Autodesk Inventor part; units mm, degrees
(part 2 of 4)
  spline S23 degree 5 poles (-0.775, -5.2999) (-0.7753, -5.3017) (-0.7759, -5.3054) (-0.7769, -5.3109) (-0.7785, -5.3181) (-0.7807, -5.3272) (-0.7831, -5.3361) (-0.7857, -5.3451) (-0.7884, -5.354) (-0.7911, -5.363) (-0.7939, -5.3719) (-0.7968, -5.3808) (-0.7998, -5.3897) (-0.8029, -5.3986) (-0.8061, -5.4075) (-0.8093, -5.4163) (-0.8127, -5.4252) (-0.8162, -5.434) (-0.8197, -5.4428) (-0.8232, -5.4516) (-0.8269, -5.4604) (-0.8306, -5.4691) (-0.8343, -5.4779) (-0.8382, -5.4866) (-0.8421, -5.4954) (-0.846, -5.5041) (-0.8501, -5.5128) (-0.8541, -5.5215) (-0.8583, -5.5302) (-0.8625, -5.5388) (-0.8667, -5.5475) (-0.8711, -5.5561) (-0.8754, -5.5648) (-0.8798, -5.5734) (-0.8843, -5.582) (-0.8888, -5.5906) (-0.8934, -5.5992) (-0.898, -5.6078) (-0.9027, -5.6163) (-0.9075, -5.6249) (-0.9122, -5.6334) (-0.9171, -5.6419) (-0.9219, -5.6504) (-0.9269, -5.6589) (-0.9318, -5.6674) (-0.9369, -5.6759) (-0.9419, -5.6844) (-0.947, -5.6928) (-0.9522, -5.7013) (-0.9574, -5.7097) (-0.9627, -5.7181) (-0.968, -5.7265) (-0.9733, -5.7349) (-0.9787, -5.7433) (-0.9841, -5.7517) (-0.9896, -5.7601) (-0.9951, -5.7684) (-1.0007, -5.7767) (-1.0063, -5.7851) (-1.0119, -5.7934) (-1.0176, -5.8017) (-1.0233, -5.81) (-1.0291, -5.8183) (-1.0349, -5.8265) (-1.0408, -5.8348) (-1.0467, -5.843) (-1.0526, -5.8512) (-1.0586, -5.8595) (-1.067, -5.8709) (-1.0743, -5.8808) (-1.0804, -5.8889) (-1.0853, -5.8954) (-1.0891, -5.9003) knots 0 0 0 0 0 0 0.014286 0.028571 0.042857 0.057143 0.071429 0.085714 0.1 0.114286 0.128571 0.142857 0.157143 0.171429 0.185714 0.2 0.214286 0.228571 0.242857 0.257143 0.271429 0.285714 0.3 0.314286 0.328571 0.342857 0.357143 0.371429 0.385714 0.4 0.414286 0.428571 0.442857 0.457143 0.471429 0.485714 0.5 0.514286 0.528571 0.542857 0.557143 0.571429 0.585714 0.6 0.614286 0.628571 0.642857 0.657143 0.671429 0.685714 0.7 0.714286 0.728571 0.742857 0.757143 0.771429 0.785714 0.8 0.814286 0.828571 0.842857 0.857143 0.871429 0.885714 0.9 0.914286 0.928571 0.942857 0.957143 1 1 1 1 1 1
  line L23 (-0.7648, -5.2336) -> (-0.775, -5.2999)
  arc A24 (-0.7648, -5.2336) -> (-0.4836, -5.267) centre (0, 0) ccw
  line L24 (-0.4836, -5.267) -> (-0.4892, -5.3339)
  spline S24 degree 5 poles (-0.4892, -5.3339) (-0.4894, -5.3357) (-0.4896, -5.3394) (-0.4899, -5.345) (-0.4901, -5.3524) (-0.4901, -5.3617) (-0.4898, -5.371) (-0.4894, -5.3803) (-0.4889, -5.3896) (-0.4883, -5.399) (-0.4877, -5.4083) (-0.487, -5.4177) (-0.4862, -5.427) (-0.4852, -5.4364) (-0.4842, -5.4457) (-0.4831, -5.4551) (-0.4819, -5.4645) (-0.4806, -5.4739) (-0.4793, -5.4833) (-0.4779, -5.4926) (-0.4764, -5.502) (-0.4749, -5.5114) (-0.4733, -5.5208) (-0.4716, -5.5302) (-0.4698, -5.5396) (-0.468, -5.549) (-0.4662, -5.5584) (-0.4642, -5.5678) (-0.4622, -5.5772) (-0.4602, -5.5867) (-0.4581, -5.5961) (-0.4559, -5.6055) (-0.4537, -5.6149) (-0.4514, -5.6243) (-0.4491, -5.6337) (-0.4467, -5.6432) (-0.4443, -5.6526) (-0.4418, -5.662) (-0.4392, -5.6714) (-0.4366, -5.6808) (-0.434, -5.6903) (-0.4313, -5.6997) (-0.4286, -5.7091) (-0.4258, -5.7185) (-0.4229, -5.7279) (-0.42, -5.7374) (-0.4171, -5.7468) (-0.4141, -5.7562) (-0.4111, -5.7656) (-0.408, -5.775) (-0.4048, -5.7845) (-0.4017, -5.7939) (-0.3984, -5.8033) (-0.3952, -5.8127) (-0.3918, -5.8221) (-0.3885, -5.8315) (-0.3851, -5.8409) (-0.3816, -5.8503) (-0.3781, -5.8598) (-0.3746, -5.8692) (-0.371, -5.8786) (-0.3674, -5.888) (-0.3637, -5.8974) (-0.36, -5.9068) (-0.3563, -5.9161) (-0.3525, -5.9255) (-0.3486, -5.9349) (-0.3447, -5.9443) (-0.3392, -5.9575) (-0.3345, -5.9687) (-0.3304, -5.9781) (-0.3272, -5.9856) (-0.3247, -5.9912) knots 0 0 0 0 0 0 0.014286 0.028571 0.042857 0.057143 0.071429 0.085714 0.1 0.114286 0.128571 0.142857 0.157143 0.171429 0.185714 0.2 0.214286 0.228571 0.242857 0.257143 0.271429 0.285714 0.3 0.314286 0.328571 0.342857 0.357143 0.371429 0.385714 0.4 0.414286 0.428571 0.442857 0.457143 0.471429 0.485714 0.5 0.514286 0.528571 0.542857 0.557143 0.571429 0.585714 0.6 0.614286 0.628571 0.642857 0.657143 0.671429 0.685714 0.7 0.714286 0.728571 0.742857 0.757143 0.771429 0.785714 0.8 0.814286 0.828571 0.842857 0.857143 0.871429 0.885714 0.9 0.914286 0.928571 0.942857 0.957143 1 1 1 1 1 1
  arc A25 (-0.3247, -5.9912) -> (-0.103, -5.9991) centre (0, 0) ccw
  spline S25 degree 5 poles (0.1079, -5.3552) (0.1079, -5.357) (0.1079, -5.3607) (0.1078, -5.3663) (0.1075, -5.3737) (0.1068, -5.383) (0.1059, -5.3922) (0.1048, -5.4015) (0.1036, -5.4108) (0.1024, -5.42) (0.1011, -5.4293) (0.0997, -5.4386) (0.0982, -5.4479) (0.0966, -5.4571) (0.095, -5.4664) (0.0932, -5.4757) (0.0913, -5.4849) (0.0894, -5.4942) (0.0874, -5.5035) (0.0853, -5.5127) (0.0831, -5.522) (0.0809, -5.5312) (0.0787, -5.5405) (0.0763, -5.5498) (0.0739, -5.559) (0.0714, -5.5683) (0.0689, -5.5775) (0.0663, -5.5868) (0.0636, -5.596) (0.0609, -5.6052) (0.0582, -5.6145) (0.0553, -5.6237) (0.0525, -5.633) (0.0495, -5.6422) (0.0465, -5.6514) (0.0435, -5.6606) (0.0404, -5.6699) (0.0372, -5.6791) (0.034, -5.6883) (0.0307, -5.6975) (0.0274, -5.7067) (0.0241, -5.7159) (0.0207, -5.7251) (0.0172, -5.7343) (0.0137, -5.7435) (0.0101, -5.7527) (0.0065, -5.7619) (0.0029, -5.7711) (-0.0008, -5.7803) (-0.0046, -5.7894) (-0.0084, -5.7986) (-0.0122, -5.8078) (-0.0161, -5.8169) (-0.02, -5.8261) (-0.024, -5.8352) (-0.028, -5.8444) (-0.0321, -5.8535) (-0.0362, -5.8627) (-0.0404, -5.8718) (-0.0446, -5.8809) (-0.0488, -5.8901) (-0.0531, -5.8992) (-0.0574, -5.9083) (-0.0618, -5.9174) (-0.0662, -5.9265) (-0.0707, -5.9356) (-0.0752, -5.9447) (-0.0797, -5.9538) (-0.0861, -5.9665) (-0.0917, -5.9774) (-0.0964, -5.9864) (-0.1002, -5.9937) (-0.103, -5.9991) knots 0 0 0 0 0 0 0.014286 0.028571 0.042857 0.057143 0.071429 0.085714 0.1 0.114286 0.128571 0.142857 0.157143 0.171429 0.185714 0.2 0.214286 0.228571 0.242857 0.257143 0.271429 0.285714 0.3 0.314286 0.328571 0.342857 0.357143 0.371429 0.385714 0.4 0.414286 0.428571 0.442857 0.457143 0.471429 0.485714 0.5 0.514286 0.528571 0.542857 0.557143 0.571429 0.585714 0.6 0.614286 0.628571 0.642857 0.657143 0.671429 0.685714 0.7 0.714286 0.728571 0.742857 0.757143 0.771429 0.785714 0.8 0.814286 0.828571 0.842857 0.857143 0.871429 0.885714 0.9 0.914286 0.928571 0.942857 0.957143 1 1 1 1 1 1
  line L25 (0.107, -5.2881) -> (0.1079, -5.3552)
  arc A26 (0.107, -5.2881) -> (0.39, -5.2748) centre (0, 0) ccw
  line L26 (0.39, -5.2748) -> (0.3954, -5.3416)
  spline S26 degree 5 poles (0.3954, -5.3416) (0.3955, -5.3435) (0.3959, -5.3472) (0.3965, -5.3527) (0.3975, -5.3601) (0.3991, -5.3692) (0.4009, -5.3784) (0.4029, -5.3875) (0.4049, -5.3966) (0.407, -5.4057) (0.4092, -5.4148) (0.4114, -5.4239) (0.4137, -5.433) (0.4162, -5.4421) (0.4187, -5.4512) (0.4214, -5.4602) (0.4241, -5.4693) (0.4269, -5.4783) (0.4298, -5.4874) (0.4327, -5.4964) (0.4357, -5.5054) (0.4388, -5.5144) (0.4419, -5.5234) (0.4451, -5.5324) (0.4484, -5.5414) (0.4517, -5.5504) (0.4551, -5.5593) (0.4585, -5.5683) (0.4621, -5.5773) (0.4656, -5.5862) (0.4693, -5.5951) (0.4729, -5.6041) (0.4767, -5.613) (0.4805, -5.6219) (0.4843, -5.6308) (0.4882, -5.6397) (0.4922, -5.6486) (0.4962, -5.6575) (0.5002, -5.6664) (0.5044, -5.6752) (0.5085, -5.6841) (0.5127, -5.6929) (0.517, -5.7018) (0.5213, -5.7106) (0.5256, -5.7194) (0.53, -5.7282) (0.5345, -5.7371) (0.539, -5.7459) (0.5435, -5.7546) (0.5481, -5.7634) (0.5528, -5.7722) (0.5575, -5.781) (0.5622, -5.7897) (0.567, -5.7985) (0.5718, -5.8072) (0.5766, -5.8159) (0.5816, -5.8247) (0.5865, -5.8334) (0.5915, -5.8421) (0.5965, -5.8508) (0.6016, -5.8594) (0.6067, -5.8681) (0.6119, -5.8768) (0.6171, -5.8854) (0.6224, -5.8941) (0.6277, -5.9027) (0.633, -5.9114) (0.6384, -5.92) (0.646, -5.932) (0.6525, -5.9424) (0.658, -5.9509) (0.6625, -5.9578) (0.6659, -5.9629) knots 0 0 0 0 0 0 0.014286 0.028571 0.042857 0.057143 0.071429 0.085714 0.1 0.114286 0.128571 0.142857 0.157143 0.171429 0.185714 0.2 0.214286 0.228571 0.242857 0.257143 0.271429 0.285714 0.3 0.314286 0.328571 0.342857 0.357143 0.371429 0.385714 0.4 0.414286 0.428571 0.442857 0.457143 0.471429 0.485714 0.5 0.514286 0.528571 0.542857 0.557143 0.571429 0.585714 0.6 0.614286 0.628571 0.642857 0.657143 0.671429 0.685714 0.7 0.714286 0.728571 0.742857 0.757143 0.771429 0.785714 0.8 0.814286 0.828571 0.842857 0.857143 0.871429 0.885714 0.9 0.914286 0.928571 0.942857 0.957143 1 1 1 1 1 1
  arc A27 (0.6659, -5.9629) -> (0.8858, -5.9343) centre (0, 0) ccw
  spline S27 degree 5 poles (0.9879, -5.2644) (0.9882, -5.2662) (0.9888, -5.2699) (0.9896, -5.2754) (0.9905, -5.2828) (0.9913, -5.292) (0.9919, -5.3013) (0.9924, -5.3106) (0.9928, -5.3199) (0.9931, -5.3293) (0.9933, -5.3386) (0.9935, -5.348) (0.9936, -5.3574) (0.9935, -5.3668) (0.9934, -5.3762) (0.9932, -5.3857) (0.9929, -5.3951) (0.9925, -5.4046) (0.992, -5.414) (0.9915, -5.4235) (0.9909, -5.433) (0.9902, -5.4425) (0.9895, -5.452) (0.9887, -5.4615) (0.9879, -5.471) (0.987, -5.4806) (0.986, -5.4901) (0.985, -5.4997) (0.9839, -5.5092) (0.9827, -5.5188) (0.9815, -5.5283) (0.9802, -5.5379) (0.9789, -5.5475) (0.9775, -5.5571) (0.9761, -5.5667) (0.9746, -5.5763) (0.973, -5.5859) (0.9715, -5.5955) (0.9698, -5.6051) (0.9681, -5.6147) (0.9664, -5.6244) (0.9646, -5.634) (0.9627, -5.6436) (0.9608, -5.6533) (0.9589, -5.6629) (0.9569, -5.6726) (0.9548, -5.6822) (0.9527, -5.6919) (0.9506, -5.7016) (0.9484, -5.7112) (0.9462, -5.7209) (0.9439, -5.7306) (0.9416, -5.7402) (0.9392, -5.7499) (0.9368, -5.7596) (0.9343, -5.7693) (0.9318, -5.779) (0.9293, -5.7887) (0.9267, -5.7984) (0.924, -5.8081) (0.9213, -5.8178) (0.9186, -5.8275) (0.9158, -5.8372) (0.913, -5.8469) (0.9102, -5.8566) (0.9073, -5.8663) (0.9043, -5.876) (0.9013, -5.8857) (0.8971, -5.8993) (0.8934, -5.9109) (0.8903, -5.9207) (0.8877, -5.9284) (0.8858, -5.9343) knots 0 0 0 0 0 0 0.014286 0.028571 0.042857 0.057143 0.071429 0.085714 0.1 0.114286 0.128571 0.142857 0.157143 0.171429 0.185714 0.2 0.214286 0.228571 0.242857 0.257143 0.271429 0.285714 0.3 0.314286 0.328571 0.342857 0.357143 0.371429 0.385714 0.4 0.414286 0.428571 0.442857 0.457143 0.471429 0.485714 0.5 0.514286 0.528571 0.542857 0.557143 0.571429 0.585714 0.6 0.614286 0.628571 0.642857 0.657143 0.671429 0.685714 0.7 0.714286 0.728571 0.742857 0.757143 0.771429 0.785714 0.8 0.814286 0.828571 0.842857 0.857143 0.871429 0.885714 0.9 0.914286 0.928571 0.942857 0.957143 1 1 1 1 1 1
  line L27 (0.976, -5.1984) -> (0.9879, -5.2644)
  arc A28 (0.976, -5.1984) -> (1.2528, -5.1387) centre (0, 0) ccw
  line L28 (1.2528, -5.1387) -> (1.2692, -5.2037)
  spline S28 degree 5 poles (1.2692, -5.2037) (1.2697, -5.2055) (1.2706, -5.2091) (1.2721, -5.2145) (1.2744, -5.2216) (1.2774, -5.2303) (1.2807, -5.239) (1.2841, -5.2477) (1.2876, -5.2563) (1.2912, -5.265) (1.2948, -5.2736) (1.2985, -5.2822) (1.3023, -5.2908) (1.3062, -5.2994) (1.3102, -5.3079) (1.3143, -5.3164) (1.3185, -5.3249) (1.3228, -5.3333) (1.3271, -5.3418) (1.3315, -5.3502) (1.3359, -5.3586) (1.3404, -5.367) (1.345, -5.3753) (1.3496, -5.3837) (1.3543, -5.392) (1.3591, -5.4003) (1.3639, -5.4086) (1.3688, -5.4169) (1.3737, -5.4251) (1.3787, -5.4334) (1.3838, -5.4416) (1.3889, -5.4498) (1.394, -5.458) (1.3993, -5.4662) (1.4045, -5.4743) (1.4098, -5.4824) (1.4152, -5.4906) (1.4206, -5.4987) (1.4261, -5.5067) (1.4316, -5.5148) (1.4371, -5.5229) (1.4428, -5.5309) (1.4484, -5.5389) (1.4541, -5.5469) (1.4599, -5.5549) (1.4657, -5.5629) (1.4715, -5.5708) (1.4774, -5.5788) (1.4833, -5.5867) (1.4893, -5.5946) (1.4953, -5.6025) (1.5014, -5.6104) (1.5075, -5.6182) (1.5136, -5.6261) (1.5198, -5.6339) (1.5261, -5.6417) (1.5323, -5.6495) (1.5387, -5.6573) (1.545, -5.665) (1.5514, -5.6728) (1.5579, -5.6805) (1.5643, -5.6882) (1.5709, -5.6959) (1.5774, -5.7036) (1.584, -5.7113) (1.5907, -5.7189) (1.5973, -5.7266) (1.6041, -5.7342) (1.6135, -5.7448) (1.6217, -5.7539) (1.6286, -5.7615) (1.6341, -5.7675) (1.6382, -5.772) knots 0 0 0 0 0 0 0.014286 0.028571 0.042857 0.057143 0.071429 0.085714 0.1 0.114286 0.128571 0.142857 0.157143 0.171429 0.185714 0.2 0.214286 0.228571 0.242857 0.257143 0.271429 0.285714 0.3 0.314286 0.328571 0.342857 0.357143 0.371429 0.385714 0.4 0.414286 0.428571 0.442857 0.457143 0.471429 0.485714 0.5 0.514286 0.528571 0.542857 0.557143 0.571429 0.585714 0.6 0.614286 0.628571 0.642857 0.657143 0.671429 0.685714 0.7 0.714286 0.728571 0.742857 0.757143 0.771429 0.785714 0.8 0.814286 0.828571 0.842857 0.857143 0.871429 0.885714 0.9 0.914286 0.928571 0.942857 0.957143 1 1 1 1 1 1
  arc A29 (1.6382, -5.772) -> (1.8505, -5.7075) centre (0, 0) ccw
  spline S29 degree 5 poles (1.8409, -5.03) (1.8415, -5.0317) (1.8427, -5.0352) (1.8444, -5.0405) (1.8465, -5.0477) (1.8489, -5.0567) (1.851, -5.0657) (1.853, -5.0748) (1.8549, -5.084) (1.8567, -5.0931) (1.8585, -5.1023) (1.8602, -5.1115) (1.8618, -5.1208) (1.8633, -5.1301) (1.8648, -5.1394) (1.8661, -5.1487) (1.8673, -5.1581) (1.8685, -5.1675) (1.8696, -5.1769) (1.8706, -5.1863) (1.8716, -5.1958) (1.8725, -5.2053) (1.8734, -5.2148) (1.8742, -5.2243) (1.8749, -5.2338) (1.8756, -5.2434) (1.8762, -5.2529) (1.8767, -5.2625) (1.8772, -5.2721) (1.8777, -5.2818) (1.878, -5.2914) (1.8784, -5.301) (1.8786, -5.3107) (1.8788, -5.3204) (1.879, -5.3301) (1.8791, -5.3398) (1.8792, -5.3495) (1.8792, -5.3593) (1.8791, -5.3691) (1.8791, -5.3788) (1.8789, -5.3886) (1.8787, -5.3984) (1.8785, -5.4082) (1.8782, -5.418) (1.8779, -5.4279) (1.8775, -5.4377) (1.8771, -5.4476) (1.8766, -5.4575) (1.8761, -5.4673) (1.8755, -5.4772) (1.8749, -5.4871) (1.8742, -5.497) (1.8735, -5.507) (1.8728, -5.5169) (1.872, -5.5269) (1.8712, -5.5368) (1.8703, -5.5468) (1.8694, -5.5568) (1.8684, -5.5668) (1.8674, -5.5768) (1.8663, -5.5868) (1.8652, -5.5968) (1.8641, -5.6068) (1.8629, -5.6168) (1.8617, -5.6269) (1.8605, -5.6369) (1.8591, -5.647) (1.8578, -5.6571) (1.8559, -5.6712) (1.8541, -5.6833) (1.8526, -5.6934) (1.8514, -5.7015) (1.8505, -5.7075) knots 0 0 0 0 0 0 0.014286 0.028571 0.042857 0.057143 0.071429 0.085714 0.1 0.114286 0.128571 0.142857 0.157143 0.171429 0.185714 0.2 0.214286 0.228571 0.242857 0.257143 0.271429 0.285714 0.3 0.314286 0.328571 0.342857 0.357143 0.371429 0.385714 0.4 0.414286 0.428571 0.442857 0.457143 0.471429 0.485714 0.5 0.514286 0.528571 0.542857 0.557143 0.571429 0.585714 0.6 0.614286 0.628571 0.642857 0.657143 0.671429 0.685714 0.7 0.714286 0.728571 0.742857 0.757143 0.771429 0.785714 0.8 0.814286 0.828571 0.842857 0.857143 0.871429 0.885714 0.9 0.914286 0.928571 0.942857 0.957143 1 1 1 1 1 1
  line L29 (1.8183, -4.9668) -> (1.8409, -5.03)
  arc A30 (1.8183, -4.9668) -> (2.0816, -4.8624) centre (0, 0) ccw
  line L30 (2.0816, -4.8624) -> (2.1084, -4.9238)
  spline S30 degree 5 poles (2.1084, -4.9238) (2.1091, -4.9255) (2.1107, -4.9289) (2.113, -4.934) (2.1164, -4.9406) (2.1209, -4.9487) (2.1255, -4.9568) (2.1303, -4.9648) (2.1352, -4.9727) (2.1402, -4.9807) (2.1452, -4.9886) (2.1503, -4.9965) (2.1554, -5.0043) (2.1607, -5.0121) (2.166, -5.0199) (2.1715, -5.0276) (2.177, -5.0352) (2.1826, -5.0429) (2.1882, -5.0505) (2.1939, -5.0581) (2.1997, -5.0656) (2.2055, -5.0732) (2.2114, -5.0807) (2.2174, -5.0881) (2.2234, -5.0956) (2.2294, -5.103) (2.2356, -5.1104) (2.2417, -5.1177) (2.248, -5.125) (2.2542, -5.1323) (2.2606, -5.1396) (2.267, -5.1469) (2.2734, -5.1541) (2.2799, -5.1613) (2.2864, -5.1685) (2.293, -5.1756) (2.2996, -5.1827) (2.3063, -5.1898) (2.313, -5.1969) (2.3198, -5.204) (2.3266, -5.211) (2.3334, -5.218) (2.3403, -5.225) (2.3473, -5.2319) (2.3543, -5.2389) (2.3613, -5.2458) (2.3684, -5.2527) (2.3755, -5.2595) (2.3826, -5.2664) (2.3898, -5.2732) (2.3971, -5.28) (2.4043, -5.2867) (2.4116, -5.2935) (2.419, -5.3002) (2.4264, -5.3069) (2.4338, -5.3136) (2.4413, -5.3202) (2.4488, -5.3269) (2.4564, -5.3335) (2.464, -5.3401) (2.4716, -5.3466) (2.4792, -5.3532) (2.4869, -5.3597) (2.4947, -5.3662) (2.5025, -5.3727) (2.5103, -5.3791) (2.5181, -5.3855) (2.526, -5.3919) (2.5371, -5.4009) (2.5466, -5.4085) (2.5547, -5.4148) (2.5611, -5.4199) (2.5659, -5.4236) knots 0 0 0 0 0 0 0.014286 0.028571 0.042857 0.057143 0.071429 0.085714 0.1 0.114286 0.128571 0.142857 0.157143 0.171429 0.185714 0.2 0.214286 0.228571 0.242857 0.257143 0.271429 0.285714 0.3 0.314286 0.328571 0.342857 0.357143 0.371429 0.385714 0.4 0.414286 0.428571 0.442857 0.457143 0.471429 0.485714 0.5 0.514286 0.528571 0.542857 0.557143 0.571429 0.585714 0.6 0.614286 0.628571 0.642857 0.657143 0.671429 0.685714 0.7 0.714286 0.728571 0.742857 0.757143 0.771429 0.785714 0.8 0.814286 0.828571 0.842857 0.857143 0.871429 0.885714 0.9 0.914286 0.928571 0.942857 0.957143 1 1 1 1 1 1
  arc A31 (2.5659, -5.4236) -> (2.7646, -5.3251) centre (0, 0) ccw
  spline S31 degree 5 poles (2.6437, -4.6584) (2.6446, -4.66) (2.6464, -4.6633) (2.6489, -4.6682) (2.6522, -4.6749) (2.6559, -4.6834) (2.6595, -4.692) (2.663, -4.7006) (2.6664, -4.7093) (2.6697, -4.7181) (2.6729, -4.7268) (2.6762, -4.7356) (2.6793, -4.7445) (2.6823, -4.7534) (2.6852, -4.7624) (2.6881, -4.7714) (2.6909, -4.7804) (2.6936, -4.7895) (2.6962, -4.7986) (2.6988, -4.8077) (2.7013, -4.8169) (2.7038, -4.8261) (2.7062, -4.8353) (2.7085, -4.8445) (2.7108, -4.8538) (2.713, -4.8631) (2.7152, -4.8725) (2.7173, -4.8819) (2.7194, -4.8912) (2.7214, -4.9007) (2.7234, -4.9101) (2.7253, -4.9196) (2.7271, -4.9291) (2.7289, -4.9386) (2.7307, -4.9481) (2.7324, -4.9577) (2.7341, -4.9673) (2.7357, -4.9769) (2.7372, -4.9865) (2.7388, -4.9962) (2.7402, -5.0059) (2.7417, -5.0155) (2.743, -5.0253) (2.7444, -5.035) (2.7457, -5.0448) (2.7469, -5.0545) (2.7481, -5.0643) (2.7493, -5.0741) (2.7504, -5.084) (2.7514, -5.0938) (2.7525, -5.1037) (2.7535, -5.1136) (2.7544, -5.1235) (2.7553, -5.1334) (2.7562, -5.1434) (2.757, -5.1533) (2.7577, -5.1633) (2.7585, -5.1733) (2.7592, -5.1833) (2.7598, -5.1933) (2.7604, -5.2034) (2.761, -5.2134) (2.7615, -5.2235) (2.762, -5.2336) (2.7625, -5.2437) (2.7629, -5.2538) (2.7633, -5.264) (2.7636, -5.2741) (2.764, -5.2884) (2.7643, -5.3006) (2.7645, -5.3108) (2.7646, -5.319) (2.7646, -5.3251) knots 0 0 0 0 0 0 0.014286 0.028571 0.042857 0.057143 0.071429 0.085714 0.1 0.114286 0.128571 0.142857 0.157143 0.171429 0.185714 0.2 0.214286 0.228571 0.242857 0.257143 0.271429 0.285714 0.3 0.314286 0.328571 0.342857 0.357143 0.371429 0.385714 0.4 0.414286 0.428571 0.442857 0.457143 0.471429 0.485714 0.5 0.514286 0.528571 0.542857 0.557143 0.571429 0.585714 0.6 0.614286 0.628571 0.642857 0.657143 0.671429 0.685714 0.7 0.714286 0.728571 0.742857 0.757143 0.771429 0.785714 0.8 0.814286 0.828571 0.842857 0.857143 0.871429 0.885714 0.9 0.914286 0.928571 0.942857 0.957143 1 1 1 1 1 1
  line L31 (2.611, -4.5998) -> (2.6437, -4.6584)
  arc A32 (2.611, -4.5998) -> (2.8535, -4.4534) centre (0, 0) ccw
  line L32 (2.8535, -4.4534) -> (2.8901, -4.5096)
  spline S32 degree 5 poles (2.8901, -4.5096) (2.8911, -4.5112) (2.8932, -4.5143) (2.8963, -4.5189) (2.9007, -4.5249) (2.9065, -4.5322) (2.9124, -4.5393) (2.9185, -4.5464) (2.9246, -4.5534) (2.9308, -4.5605) (2.937, -4.5674) (2.9433, -4.5744) (2.9497, -4.5813) (2.9562, -4.5881) (2.9627, -4.5949) (2.9694, -4.6016) (2.9761, -4.6082) (2.9828, -4.6149) (2.9897, -4.6214) (2.9965, -4.628) (3.0035, -4.6345) (3.0105, -4.6409) (3.0175, -4.6474) (3.0246, -4.6538) (3.0317, -4.6601) (3.0389, -4.6664) (3.0462, -4.6727) (3.0535, -4.6789) (3.0609, -4.6851) (3.0683, -4.6913) (3.0757, -4.6974) (3.0832, -4.7035) (3.0907, -4.7096) (3.0983, -4.7156) (3.1059, -4.7216) (3.1136, -4.7276) (3.1213, -4.7336) (3.129, -4.7395) (3.1368, -4.7453) (3.1447, -4.7512) (3.1525, -4.757) (3.1605, -4.7628) (3.1684, -4.7685) (3.1764, -4.7742) (3.1844, -4.7799) (3.1925, -4.7856) (3.2006, -4.7912) (3.2088, -4.7968) (3.2169, -4.8024) (3.2252, -4.8079) (3.2334, -4.8134) (3.2417, -4.8189) (3.25, -4.8243) (3.2584, -4.8298) (3.2668, -4.8351) (3.2752, -4.8405) (3.2837, -4.8458) (3.2922, -4.8511) (3.3007, -4.8564) (3.3093, -4.8617) (3.3179, -4.8669) (3.3265, -4.8721) (3.3352, -4.8772) (3.3439, -4.8824) (3.3526, -4.8875) (3.3614, -4.8926) (3.3702, -4.8976) (3.379, -4.9026) (3.3914, -4.9096) (3.4021, -4.9156) (3.4111, -4.9205) (3.4183, -4.9244) (3.4237, -4.9273) knots 0 0 0 0 0 0 0.014286 0.028571 0.042857 0.057143 0.071429 0.085714 0.1 0.114286 0.128571 0.142857 0.157143 0.171429 0.185714 0.2 0.214286 0.228571 0.242857 0.257143 0.271429 0.285714 0.3 0.314286 0.328571 0.342857 0.357143 0.371429 0.385714 0.4 0.414286 0.428571 0.442857 0.457143 0.471429 0.485714 0.5 0.514286 0.528571 0.542857 0.557143 0.571429 0.585714 0.6 0.614286 0.628571 0.642857 0.657143 0.671429 0.685714 0.7 0.714286 0.728571 0.742857 0.757143 0.771429 0.785714 0.8 0.814286 0.828571 0.842857 0.857143 0.871429 0.885714 0.9 0.914286 0.928571 0.942857 0.957143 1 1 1 1 1 1
  arc A33 (3.4237, -4.9273) -> (3.6034, -4.7974) centre (0, 0) ccw
  spline S33 degree 5 poles (3.3744, -4.1597) (3.3755, -4.1612) (3.3778, -4.1641) (3.3812, -4.1685) (3.3855, -4.1746) (3.3906, -4.1824) (3.3955, -4.1902) (3.4004, -4.1982) (3.4051, -4.2062) (3.4098, -4.2143) (3.4145, -4.2224) (3.4191, -4.2306) (3.4237, -4.2388) (3.4281, -4.2471) (3.4325, -4.2554) (3.4368, -4.2638) (3.441, -4.2723) (3.4451, -4.2808) (3.4492, -4.2894) (3.4533, -4.2979) (3.4573, -4.3066) (3.4612, -4.3152) (3.4651, -4.3239) (3.469, -4.3327) (3.4727, -4.3414) (3.4765, -4.3503) (3.4802, -4.3591) (3.4838, -4.368) (3.4874, -4.3769) (3.4909, -4.3859) (3.4944, -4.3949) (3.4978, -4.4039) (3.5012, -4.413) (3.5046, -4.4221) (3.5079, -4.4312) (3.5111, -4.4403) (3.5144, -4.4495) (3.5175, -4.4587) (3.5207, -4.468) (3.5237, -4.4773) (3.5268, -4.4866) (3.5298, -4.4959) (3.5328, -4.5052) (3.5357, -4.5146) (3.5386, -4.524) (3.5414, -4.5335) (3.5442, -4.5429) (3.5469, -4.5524) (3.5497, -4.5619) (3.5523, -4.5715) (3.555, -4.581) (3.5576, -4.5906) (3.5601, -4.6003) (3.5627, -4.6099) (3.5651, -4.6196) (3.5676, -4.6293) (3.57, -4.639) (3.5724, -4.6487) (3.5747, -4.6585) (3.577, -4.6682) (3.5792, -4.6781) (3.5815, -4.6879) (3.5836, -4.6977) (3.5858, -4.7076) (3.5879, -4.7175) (3.59, -4.7274) (3.592, -4.7374) (3.594, -4.7473) (3.5967, -4.7613) (3.599, -4.7733) (3.6009, -4.7833) (3.6023, -4.7914) (3.6034, -4.7974) knots 0 0 0 0 0 0 0.014286 0.028571 0.042857 0.057143 0.071429 0.085714 0.1 0.114286 0.128571 0.142857 0.157143 0.171429 0.185714 0.2 0.214286 0.228571 0.242857 0.257143 0.271429 0.285714 0.3 0.314286 0.328571 0.342857 0.357143 0.371429 0.385714 0.4 0.414286 0.428571 0.442857 0.457143 0.471429 0.485714 0.5 0.514286 0.528571 0.542857 0.557143 0.571429 0.585714 0.6 0.614286 0.628571 0.642857 0.657143 0.671429 0.685714 0.7 0.714286 0.728571 0.742857 0.757143 0.771429 0.785714 0.8 0.814286 0.828571 0.842857 0.857143 0.871429 0.885714 0.9 0.914286 0.928571 0.942857 0.957143 1 1 1 1 1 1
  line L33 (3.3325, -4.1073) -> (3.3744, -4.1597)
  arc A34 (3.3325, -4.1073) -> (3.5476, -3.923) centre (0, 0) ccw
  line L34 (3.5476, -3.923) -> (3.5929, -3.9724)
  spline S34 degree 5 poles (3.5929, -3.9724) (3.5942, -3.9738) (3.5967, -3.9765) (3.6006, -3.9805) (3.6059, -3.9857) (3.6128, -3.9919) (3.6198, -3.998) (3.627, -4.004) (3.6342, -4.01) (3.6414, -4.0159) (3.6487, -4.0217) (3.6561, -4.0275) (3.6635, -4.0333) (3.671, -4.039) (3.6786, -4.0446) (3.6863, -4.0501) (3.694, -4.0556) (3.7017, -4.061) (3.7095, -4.0663) (3.7174, -4.0716) (3.7253, -4.0769) (3.7333, -4.0821) (3.7413, -4.0873) (3.7493, -4.0925) (3.7574, -4.0976) (3.7656, -4.1026) (3.7738, -4.1076) (3.782, -4.1125) (3.7903, -4.1174) (3.7986, -4.1223) (3.8069, -4.1271) (3.8153, -4.1319) (3.8237, -4.1367) (3.8322, -4.1414) (3.8407, -4.146) (3.8493, -4.1507) (3.8578, -4.1552) (3.8665, -4.1598) (3.8751, -4.1643) (3.8838, -4.1688) (3.8925, -4.1732) (3.9013, -4.1776) (3.9101, -4.182) (3.9189, -4.1863) (3.9278, -4.1906) (3.9366, -4.1948) (3.9456, -4.199) (3.9545, -4.2032) (3.9635, -4.2074) (3.9725, -4.2115) (3.9816, -4.2156) (3.9907, -4.2196) (3.9998, -4.2236) (4.0089, -4.2276) (4.0181, -4.2315) (4.0273, -4.2354) (4.0365, -4.2393) (4.0458, -4.2431) (4.0551, -4.2469) (4.0644, -4.2507) (4.0737, -4.2544) (4.0831, -4.2581) (4.0925, -4.2618) (4.1019, -4.2654) (4.1114, -4.269) (4.1208, -4.2726) (4.1304, -4.2761) (4.1399, -4.2796) (4.1533, -4.2845) (4.1648, -4.2886) (4.1744, -4.2919) (4.1822, -4.2946) (4.188, -4.2966) knots 0 0 0 0 0 0 0.014286 0.028571 0.042857 0.057143 0.071429 0.085714 0.1 0.114286 0.128571 0.142857 0.157143 0.171429 0.185714 0.2 0.214286 0.228571 0.242857 0.257143 0.271429 0.285714 0.3 0.314286 0.328571 0.342857 0.357143 0.371429 0.385714 0.4 0.414286 0.428571 0.442857 0.457143 0.471429 0.485714 0.5 0.514286 0.528571 0.542857 0.557143 0.571429 0.585714 0.6 0.614286 0.628571 0.642857 0.657143 0.671429 0.685714 0.7 0.714286 0.728571 0.742857 0.757143 0.771429 0.785714 0.8 0.814286 0.828571 0.842857 0.857143 0.871429 0.885714 0.9 0.914286 0.928571 0.942857 0.957143 1 1 1 1 1 1
  arc A35 (4.188, -4.2966) -> (4.3439, -4.1389) centre (0, 0) ccw
  spline S35 degree 5 poles (4.013, -3.5476) (4.0144, -3.5488) (4.0171, -3.5513) (4.0212, -3.5552) (4.0264, -3.5604) (4.0327, -3.5672) (4.0389, -3.5742) (4.045, -3.5813) (4.051, -3.5884) (4.057, -3.5956) (4.0629, -3.6028) (4.0688, -3.6101) (4.0746, -3.6175) (4.0804, -3.6249) (4.0861, -3.6324) (4.0917, -3.64) (4.0972, -3.6477) (4.1027, -3.6554) (4.1082, -3.6631) (4.1136, -3.6709) (4.119, -3.6788) (4.1243, -3.6867) (4.1296, -3.6946) (4.1348, -3.7026) (4.14, -3.7106) (4.1451, -3.7187) (4.1502, -3.7269) (4.1552, -3.735) (4.1602, -3.7432) (4.1652, -3.7515) (4.1701, -3.7598) (4.175, -3.7681) (4.1798, -3.7765) (4.1846, -3.7849) (4.1894, -3.7934) (4.1941, -3.8019) (4.1988, -3.8104) (4.2034, -3.819) (4.208, -3.8276) (4.2126, -3.8362) (4.2172, -3.8449) (4.2216, -3.8536) (4.2261, -3.8623) (4.2305, -3.8711) (4.2349, -3.8799) (4.2393, -3.8887) (4.2436, -3.8976) (4.2479, -3.9065) (4.2521, -3.9155) (4.2563, -3.9244) (4.2605, -3.9334) (4.2646, -3.9425) (4.2688, -3.9515) (4.2728, -3.9606) (4.2769, -3.9698) (4.2809, -3.9789) (4.2848, -3.9881) (4.2888, -3.9973) (4.2927, -4.0066) (4.2966, -4.0158) (4.3004, -4.0251) (4.3042, -4.0345) (4.308, -4.0438) (4.3117, -4.0532) (4.3154, -4.0626) (4.3191, -4.0721) (4.3227, -4.0815) (4.3264, -4.091) (4.3314, -4.1043) (4.3356, -4.1158) (4.3391, -4.1254) (4.3418, -4.1331) (4.3439, -4.1389) knots 0 0 0 0 0 0 0.014286 0.028571 0.042857 0.057143 0.071429 0.085714 0.1 0.114286 0.128571 0.142857 0.157143 0.171429 0.185714 0.2 0.214286 0.228571 0.242857 0.257143 0.271429 0.285714 0.3 0.314286 0.328571 0.342857 0.357143 0.371429 0.385714 0.4 0.414286 0.428571 0.442857 0.457143 0.471429 0.485714 0.5 0.514286 0.528571 0.542857 0.557143 0.571429 0.585714 0.6 0.614286 0.628571 0.642857 0.657143 0.671429 0.685714 0.7 0.714286 0.728571 0.742857 0.757143 0.771429 0.785714 0.8 0.814286 0.828571 0.842857 0.857143 0.871429 0.885714 0.9 0.914286 0.928571 0.942857 0.957143 1 1 1 1 1 1
  line L35 (3.9631, -3.5028) -> (4.013, -3.5476)
  arc A36 (3.9631, -3.5028) -> (4.1449, -3.2856) centre (0, 0) ccw
  line L36 (4.1449, -3.2856) -> (4.1978, -3.3269)
  spline S36 degree 5 poles (4.1978, -3.3269) (4.1992, -3.328) (4.2022, -3.3303) (4.2067, -3.3336) (4.2128, -3.3378) (4.2206, -3.3429) (4.2285, -3.3477) (4.2365, -3.3524) (4.2446, -3.3571) (4.2528, -3.3617) (4.2609, -3.3663) (4.2691, -3.3708) (4.2774, -3.3753) (4.2858, -3.3797) (4.2941, -3.3839) (4.3026, -3.3881) (4.3111, -3.3922) (4.3197, -3.3963) (4.3283, -3.4003) (4.3369, -3.4042) (4.3455, -3.4081) (4.3543, -3.412) (4.363, -3.4158) (4.3718, -3.4195) (4.3806, -3.4232) (4.3895, -3.4268) (4.3984, -3.4304) (4.4073, -3.4339) (4.4163, -3.4374) (4.4253, -3.4409) (4.4343, -3.4442) (4.4434, -3.4476) (4.4525, -3.4509) (4.4616, -3.4541) (4.4707, -3.4573) (4.4799, -3.4605) (4.4892, -3.4636) (4.4984, -3.4667) (4.5077, -3.4697) (4.517, -3.4727) (4.5263, -3.4756) (4.5357, -3.4785) (4.5451, -3.4814) (4.5545, -3.4842) (4.5639, -3.4869) (4.5734, -3.4897) (4.5829, -3.4924) (4.5924, -3.495) (4.602, -3.4976) (4.6115, -3.5002) (4.6211, -3.5027) (4.6308, -3.5052) (4.6404, -3.5077) (4.6501, -3.5101) (4.6598, -3.5124) (4.6695, -3.5148) (4.6792, -3.5171) (4.689, -3.5193) (4.6988, -3.5215) (4.7086, -3.5237) (4.7184, -3.5259) (4.7283, -3.528) (4.7381, -3.53) (4.748, -3.5321) (4.7579, -3.5341) (4.7679, -3.536) (4.7778, -3.5379) (4.7878, -3.5398) (4.8018, -3.5424) (4.8139, -3.5446) (4.8239, -3.5463) (4.832, -3.5477) (4.8381, -3.5487) knots 0 0 0 0 0 0 0.014286 0.028571 0.042857 0.057143 0.071429 0.085714 0.1 0.114286 0.128571 0.142857 0.157143 0.171429 0.185714 0.2 0.214286 0.228571 0.242857 0.257143 0.271429 0.285714 0.3 0.314286 0.328571 0.342857 0.357143 0.371429 0.385714 0.4 0.414286 0.428571 0.442857 0.457143 0.471429 0.485714 0.5 0.514286 0.528571 0.542857 0.557143 0.571429 0.585714 0.6 0.614286 0.628571 0.642857 0.657143 0.671429 0.685714 0.7 0.714286 0.728571 0.742857 0.757143 0.771429 0.785714 0.8 0.814286 0.828571 0.842857 0.857143 0.871429 0.885714 0.9 0.914286 0.928571 0.942857 0.957143 1 1 1 1 1 1
  arc A37 (4.8381, -3.5487) -> (4.9659, -3.3675) centre (0, 0) ccw
  spline S37 degree 5 poles (4.5422, -2.8387) (4.5437, -2.8397) (4.5469, -2.8417) (4.5515, -2.8448) (4.5575, -2.8492) (4.5649, -2.8548) (4.5721, -2.8607) (4.5793, -2.8666) (4.5864, -2.8727) (4.5935, -2.8788) (4.6005, -2.8849) (4.6075, -2.8912) (4.6145, -2.8975) (4.6214, -2.9039) (4.6282, -2.9103) (4.635, -2.9169) (4.6418, -2.9235) (4.6484, -2.9302) (4.6551, -2.937) (4.6617, -2.9438) (4.6683, -2.9506) (4.6748, -2.9575) (4.6814, -2.9645) (4.6878, -2.9715) (4.6943, -2.9786) (4.7006, -2.9857) (4.707, -2.9929) (4.7133, -3.0002) (4.7196, -3.0074) (4.7259, -3.0148) (4.7321, -3.0221) (4.7383, -3.0296) (4.7444, -3.037) (4.7505, -3.0445) (4.7566, -3.0521) (4.7627, -3.0597) (4.7687, -3.0673) (4.7747, -3.075) (4.7807, -3.0827) (4.7866, -3.0905) (4.7925, -3.0983) (4.7984, -3.1062) (4.8042, -3.114) (4.81, -3.122) (4.8158, -3.1299) (4.8215, -3.1379) (4.8272, -3.146) (4.8329, -3.1541) (4.8386, -3.1622) (4.8442, -3.1703) (4.8498, -3.1785) (4.8554, -3.1868) (4.8609, -3.195) (4.8665, -3.2033) (4.8719, -3.2117) (4.8774, -3.22) (4.8828, -3.2284) (4.8882, -3.2369) (4.8936, -3.2454) (4.8989, -3.2539) (4.9043, -3.2624) (4.9096, -3.271) (4.9148, -3.2796) (4.92, -3.2882) (4.9253, -3.2969) (4.9304, -3.3056) (4.9356, -3.3144) (4.9407, -3.3231) (4.9478, -3.3355) (4.9539, -3.3461) (4.9589, -3.355) (4.9629, -3.3621) (4.9659, -3.3675) knots 0 0 0 0 0 0 0.014286 0.028571 0.042857 0.057143 0.071429 0.085714 0.1 0.114286 0.128571 0.142857 0.157143 0.171429 0.185714 0.2 0.214286 0.228571 0.242857 0.257143 0.271429 0.285714 0.3 0.314286 0.328571 0.342857 0.357143 0.371429 0.385714 0.4 0.414286 0.428571 0.442857 0.457143 0.471429 0.485714 0.5 0.514286 0.528571 0.542857 0.557143 0.571429 0.585714 0.6 0.614286 0.628571 0.642857 0.657143 0.671429 0.685714 0.7 0.714286 0.728571 0.742857 0.757143 0.771429 0.785714 0.8 0.814286 0.828571 0.842857 0.857143 0.871429 0.885714 0.9 0.914286 0.928571 0.942857 0.957143 1 1 1 1 1 1
  line L37 (4.4856, -2.8027) -> (4.5422, -2.8387)
  arc A38 (4.4856, -2.8027) -> (4.6292, -2.5586) centre (0, 0) ccw
  line L38 (4.6292, -2.5586) -> (4.6881, -2.5906)
  spline S38 degree 5 poles (4.6881, -2.5906) (4.6897, -2.5915) (4.693, -2.5932) (4.698, -2.5957) (4.7047, -2.5989) (4.7132, -2.6026) (4.7219, -2.6061) (4.7306, -2.6094) (4.7393, -2.6127) (4.7481, -2.6159) (4.7569, -2.6191) (4.7657, -2.6222) (4.7746, -2.6252) (4.7836, -2.6281) (4.7926, -2.631) (4.8016, -2.6337) (4.8107, -2.6364) (4.8198, -2.639) (4.8289, -2.6415) (4.8381, -2.644) (4.8472, -2.6464) (4.8565, -2.6488) (4.8657, -2.6511) (4.875, -2.6533) (4.8843, -2.6555) (4.8936, -2.6576) (4.903, -2.6597) (4.9124, -2.6617) (4.9218, -2.6636) (4.9313, -2.6656) (4.9407, -2.6674) (4.9502, -2.6692) (4.9597, -2.671) (4.9693, -2.6727) (4.9788, -2.6743) (4.9884, -2.6759) (4.998, -2.6775) (5.0076, -2.679) (5.0173, -2.6804) (5.027, -2.6818) (5.0367, -2.6832) (5.0464, -2.6845) (5.0561, -2.6858) (5.0658, -2.687) (5.0756, -2.6882) (5.0854, -2.6893) (5.0952, -2.6904) (5.105, -2.6915) (5.1149, -2.6925) (5.1248, -2.6934) (5.1346, -2.6943) (5.1445, -2.6952) (5.1544, -2.696) (5.1644, -2.6968) (5.1743, -2.6976) (5.1843, -2.6983) (5.1943, -2.6989) (5.2043, -2.6995) (5.2143, -2.7001) (5.2243, -2.7007) (5.2344, -2.7012) (5.2445, -2.7016) (5.2545, -2.702) (5.2646, -2.7024) (5.2747, -2.7027) (5.2849, -2.703) (5.295, -2.7033) (5.3052, -2.7035) (5.3194, -2.7037) (5.3316, -2.7039) (5.3418, -2.704) (5.35, -2.704) (5.3562, -2.704) knots 0 0 0 0 0 0 0.014286 0.028571 0.042857 0.057143 0.071429 0.085714 0.1 0.114286 0.128571 0.142857 0.157143 0.171429 0.185714 0.2 0.214286 0.228571 0.242857 0.257143 0.271429 0.285714 0.3 0.314286 0.328571 0.342857 0.357143 0.371429 0.385714 0.4 0.414286 0.428571 0.442857 0.457143 0.471429 0.485714 0.5 0.514286 0.528571 0.542857 0.557143 0.571429 0.585714 0.6 0.614286 0.628571 0.642857 0.657143 0.671429 0.685714 0.7 0.714286 0.728571 0.742857 0.757143 0.771429 0.785714 0.8 0.814286 0.828571 0.842857 0.857143 0.871429 0.885714 0.9 0.914286 0.928571 0.942857 0.957143 1 1 1 1 1 1
  arc A39 (5.3562, -2.704) -> (5.4524, -2.5042) centre (0, 0) ccw
  spline S39 degree 5 poles (4.9475, -2.0523) (4.9492, -2.0531) (4.9526, -2.0545) (4.9576, -2.0569) (4.9643, -2.0602) (4.9725, -2.0645) (4.9806, -2.0691) (4.9886, -2.0738) (4.9966, -2.0786) (5.0046, -2.0835) (5.0126, -2.0884) (5.0206, -2.0934) (5.0285, -2.0984) (5.0363, -2.1036) (5.0441, -2.1089) (5.0519, -2.1142) (5.0596, -2.1196) (5.0673, -2.1252) (5.075, -2.1307) (5.0827, -2.1363) (5.0903, -2.142) (5.0979, -2.1478) (5.1054, -2.1536) (5.113, -2.1594) (5.1205, -2.1653) (5.128, -2.1713) (5.1354, -2.1774) (5.1428, -2.1835) (5.1502, -2.1896) (5.1576, -2.1958) (5.165, -2.2021) (5.1723, -2.2083) (5.1796, -2.2147) (5.1869, -2.2211) (5.1941, -2.2275) (5.2013, -2.234) (5.2085, -2.2406) (5.2157, -2.2472) (5.2229, -2.2538) (5.23, -2.2605) (5.2371, -2.2672) (5.2442, -2.274) (5.2512, -2.2808) (5.2583, -2.2877) (5.2653, -2.2946) (5.2723, -2.3016) (5.2792, -2.3085) (5.2862, -2.3156) (5.2931, -2.3227) (5.3, -2.3298) (5.3068, -2.3369) (5.3137, -2.3441) (5.3205, -2.3514) (5.3273, -2.3586) (5.3341, -2.366) (5.3409, -2.3733) (5.3476, -2.3807) (5.3543, -2.3882) (5.361, -2.3956) (5.3677, -2.4031) (5.3743, -2.4107) (5.381, -2.4183) (5.3876, -2.4259) (5.3942, -2.4336) (5.4007, -2.4413) (5.4073, -2.449) (5.4138, -2.4568) (5.4203, -2.4646) (5.4294, -2.4756) (5.4371, -2.4851) (5.4435, -2.493) (5.4486, -2.4994) (5.4524, -2.5042) knots 0 0 0 0 0 0 0.014286 0.028571 0.042857 0.057143 0.071429 0.085714 0.1 0.114286 0.128571 0.142857 0.157143 0.171429 0.185714 0.2 0.214286 0.228571 0.242857 0.257143 0.271429 0.285714 0.3 0.314286 0.328571 0.342857 0.357143 0.371429 0.385714 0.4 0.414286 0.428571 0.442857 0.457143 0.471429 0.485714 0.5 0.514286 0.528571 0.542857 0.557143 0.571429 0.585714 0.6 0.614286 0.628571 0.642857 0.657143 0.671429 0.685714 0.7 0.714286 0.728571 0.742857 0.757143 0.771429 0.785714 0.8 0.814286 0.828571 0.842857 0.857143 0.871429 0.885714 0.9 0.914286 0.928571 0.942857 0.957143 1 1 1 1 1 1
  line L39 (4.8857, -2.0262) -> (4.9475, -2.0523)
  arc A40 (4.8857, -2.0262) -> (4.9872, -1.7617) centre (0, 0) ccw
  line L40 (4.9872, -1.7617) -> (5.0506, -1.7836)
  spline S40 degree 5 poles (5.0506, -1.7836) (5.0523, -1.7842) (5.0558, -1.7854) (5.0612, -1.7871) (5.0683, -1.7891) (5.0773, -1.7913) (5.0864, -1.7933) (5.0955, -1.7952) (5.1047, -1.797) (5.1139, -1.7987) (5.1231, -1.8004) (5.1323, -1.802) (5.1416, -1.8035) (5.1509, -1.805) (5.1602, -1.8063) (5.1696, -1.8075) (5.179, -1.8086) (5.1884, -1.8097) (5.1978, -1.8107) (5.2073, -1.8116) (5.2167, -1.8125) (5.2262, -1.8133) (5.2357, -1.814) (5.2452, -1.8147) (5.2548, -1.8154) (5.2643, -1.8159) (5.2739, -1.8164) (5.2835, -1.8168) (5.2931, -1.8172) (5.3027, -1.8175) (5.3124, -1.8178) (5.322, -1.818) (5.3317, -1.8182) (5.3414, -1.8183) (5.3511, -1.8183) (5.3608, -1.8183) (5.3705, -1.8183) (5.3803, -1.8182) (5.39, -1.818) (5.3998, -1.8178) (5.4096, -1.8176) (5.4194, -1.8173) (5.4292, -1.8169) (5.439, -1.8165) (5.4489, -1.8161) (5.4587, -1.8156) (5.4685, -1.8151) (5.4784, -1.8145) (5.4883, -1.8138) (5.4982, -1.8132) (5.5081, -1.8124) (5.518, -1.8117) (5.5279, -1.8109) (5.5378, -1.81) (5.5478, -1.8091) (5.5577, -1.8082) (5.5677, -1.8072) (5.5776, -1.8061) (5.5876, -1.805) (5.5976, -1.8039) (5.6076, -1.8028) (5.6176, -1.8016) (5.6276, -1.8003) (5.6376, -1.799) (5.6477, -1.7977) (5.6577, -1.7963) (5.6677, -1.7949) (5.6778, -1.7934) (5.6919, -1.7913) (5.704, -1.7895) (5.714, -1.7878) (5.7221, -1.7865) (5.7282, -1.7855) knots 0 0 0 0 0 0 0.014286 0.028571 0.042857 0.057143 0.071429 0.085714 0.1 0.114286 0.128571 0.142857 0.157143 0.171429 0.185714 0.2 0.214286 0.228571 0.242857 0.257143 0.271429 0.285714 0.3 0.314286 0.328571 0.342857 0.357143 0.371429 0.385714 0.4 0.414286 0.428571 0.442857 0.457143 0.471429 0.485714 0.5 0.514286 0.528571 0.542857 0.557143 0.571429 0.585714 0.6 0.614286 0.628571 0.642857 0.657143 0.671429 0.685714 0.7 0.714286 0.728571 0.742857 0.757143 0.771429 0.785714 0.8 0.814286 0.828571 0.842857 0.857143 0.871429 0.885714 0.9 0.914286 0.928571 0.942857 0.957143 1 1 1 1 1 1
  arc A41 (5.7282, -1.7855) -> (5.7902, -1.5726) centre (0, 0) ccw
  spline S41 degree 5 poles (5.2178, -1.21) (5.2196, -1.2105) (5.2232, -1.2114) (5.2286, -1.2128) (5.2357, -1.215) (5.2445, -1.2179) (5.2532, -1.2211) (5.2619, -1.2244) (5.2706, -1.2278) (5.2793, -1.2313) (5.288, -1.2348) (5.2966, -1.2385) (5.3053, -1.2422) (5.3139, -1.246) (5.3225, -1.2499) (5.331, -1.2539) (5.3395, -1.2579) (5.348, -1.2621) (5.3565, -1.2663) (5.365, -1.2706) (5.3734, -1.275) (5.3819, -1.2794) (5.3903, -1.2839) (5.3987, -1.2884) (5.4071, -1.293) (5.4154, -1.2977) (5.4238, -1.3024) (5.4321, -1.3072) (5.4404, -1.312) (5.4487, -1.3169) (5.457, -1.3219) (5.4652, -1.3269) (5.4735, -1.332) (5.4817, -1.3371) (5.4899, -1.3422) (5.4981, -1.3475) (5.5063, -1.3527) (5.5144, -1.3581) (5.5226, -1.3634) (5.5307, -1.3689) (5.5388, -1.3743) (5.5469, -1.3798) (5.555, -1.3854) (5.5631, -1.391) (5.5711, -1.3967) (5.5792, -1.4024) (5.5872, -1.4081) (5.5952, -1.4139) (5.6032, -1.4198) (5.6112, -1.4256) (5.6191, -1.4316) (5.6271, -1.4376) (5.635, -1.4436) (5.6429, -1.4496) (5.6508, -1.4557) (5.6587, -1.4619) (5.6665, -1.4681) (5.6744, -1.4743) (5.6822, -1.4806) (5.69, -1.4869) (5.6978, -1.4932) (5.7056, -1.4996) (5.7134, -1.5061) (5.7212, -1.5125) (5.7289, -1.519) (5.7366, -1.5256) (5.7443, -1.5322) (5.752, -1.5388) (5.7628, -1.5482) (5.772, -1.5562) (5.7796, -1.563) (5.7857, -1.5685) (5.7902, -1.5726) knots 0 0 0 0 0 0 0.014286 0.028571 0.042857 0.057143 0.071429 0.085714 0.1 0.114286 0.128571 0.142857 0.157143 0.171429 0.185714 0.2 0.214286 0.228571 0.242857 0.257143 0.271429 0.285714 0.3 0.314286 0.328571 0.342857 0.357143 0.371429 0.385714 0.4 0.414286 0.428571 0.442857 0.457143 0.471429 0.485714 0.5 0.514286 0.528571 0.542857 0.557143 0.571429 0.585714 0.6 0.614286 0.628571 0.642857 0.657143 0.671429 0.685714 0.7 0.714286 0.728571 0.742857 0.757143 0.771429 0.785714 0.8 0.814286 0.828571 0.842857 0.857143 0.871429 0.885714 0.9 0.914286 0.928571 0.942857 0.957143 1 1 1 1 1 1
  line L41 (5.1526, -1.1944) -> (5.2178, -1.21)
  arc A42 (5.1526, -1.1944) -> (5.2091, -0.9169) centre (0, 0) ccw
  line L42 (5.2091, -0.9169) -> (5.2752, -0.928)
  spline S42 degree 5 poles (5.2752, -0.928) (5.2771, -0.9283) (5.2808, -0.9289) (5.2863, -0.9296) (5.2937, -0.9305) (5.3029, -0.9312) (5.3122, -0.9317) (5.3215, -0.932) (5.3308, -0.9323) (5.3402, -0.9325) (5.3496, -0.9326) (5.3589, -0.9327) (5.3683, -0.9327) (5.3777, -0.9325) (5.3872, -0.9323) (5.3966, -0.9319) (5.406, -0.9315) (5.4155, -0.931) (5.4249, -0.9304) (5.4344, -0.9298) (5.4439, -0.9291) (5.4534, -0.9284) (5.4629, -0.9275) (5.4724, -0.9266) (5.4819, -0.9257) (5.4914, -0.9247) (5.501, -0.9236) (5.5105, -0.9224) (5.52, -0.9212) (5.5296, -0.9199) (5.5391, -0.9186) (5.5487, -0.9173) (5.5583, -0.9158) (5.5678, -0.9143) (5.5774, -0.9128) (5.587, -0.9112) (5.5966, -0.9095) (5.6062, -0.9078) (5.6158, -0.9061) (5.6254, -0.9043) (5.635, -0.9024) (5.6446, -0.9005) (5.6542, -0.8985) (5.6638, -0.8965) (5.6735, -0.8945) (5.6831, -0.8924) (5.6927, -0.8902) (5.7023, -0.888) (5.712, -0.8858) (5.7216, -0.8835) (5.7313, -0.8811) (5.7409, -0.8787) (5.7506, -0.8763) (5.7602, -0.8738) (5.7699, -0.8713) (5.7795, -0.8687) (5.7892, -0.8661) (5.7988, -0.8634) (5.8085, -0.8607) (5.8182, -0.858) (5.8278, -0.8552) (5.8375, -0.8524) (5.8472, -0.8495) (5.8568, -0.8466) (5.8665, -0.8436) (5.8762, -0.8406) (5.8859, -0.8375) (5.8955, -0.8344) (5.9091, -0.83) (5.9207, -0.8262) (5.9304, -0.823) (5.9381, -0.8203) (5.9439, -0.8183) knots 0 0 0 0 0 0 0.014286 0.028571 0.042857 0.057143 0.071429 0.085714 0.1 0.114286 0.128571 0.142857 0.157143 0.171429 0.185714 0.2 0.214286 0.228571 0.242857 0.257143 0.271429 0.285714 0.3 0.314286 0.328571 0.342857 0.357143 0.371429 0.385714 0.4 0.414286 0.428571 0.442857 0.457143 0.471429 0.485714 0.5 0.514286 0.528571 0.542857 0.557143 0.571429 0.585714 0.6 0.614286 0.628571 0.642857 0.657143 0.671429 0.685714 0.7 0.714286 0.728571 0.742857 0.757143 0.771429 0.785714 0.8 0.814286 0.828571 0.842857 0.857143 0.871429 0.885714 0.9 0.914286 0.928571 0.942857 0.957143 1 1 1 1 1 1
  arc A43 (5.9439, -0.8183) -> (5.9701, -0.5981) centre (0, 0) ccw
  spline S43 degree 5 poles (5.3458, -0.3347) (5.3476, -0.3348) (5.3513, -0.3351) (5.3569, -0.3357) (5.3643, -0.3366) (5.3734, -0.3381) (5.3826, -0.3398) (5.3917, -0.3416) (5.4008, -0.3436) (5.41, -0.3456) (5.4191, -0.3476) (5.4282, -0.3498) (5.4374, -0.352) (5.4465, -0.3543) (5.4556, -0.3568) (5.4647, -0.3593) (5.4737, -0.3619) (5.4828, -0.3646) (5.4919, -0.3674) (5.5009, -0.3702) (5.51, -0.3731) (5.519, -0.3761) (5.5281, -0.3791) (5.5371, -0.3822) (5.5461, -0.3854) (5.5551, -0.3886) (5.5642, -0.3919) (5.5732, -0.3953) (5.5822, -0.3987) (5.5911, -0.4022) (5.6001, -0.4057) (5.6091, -0.4093) (5.6181, -0.4129) (5.627, -0.4166) (5.636, -0.4203) (5.6449, -0.4241) (5.6538, -0.428) (5.6628, -0.4319) (5.6717, -0.4358) (5.6806, -0.4399) (5.6895, -0.4439) (5.6984, -0.448) (5.7073, -0.4522) (5.7162, -0.4564) (5.725, -0.4606) (5.7339, -0.4649) (5.7428, -0.4693) (5.7516, -0.4737) (5.7604, -0.4781) (5.7693, -0.4826) (5.7781, -0.4872) (5.7869, -0.4918) (5.7957, -0.4964) (5.8045, -0.5011) (5.8133, -0.5058) (5.8221, -0.5106) (5.8309, -0.5154) (5.8397, -0.5202) (5.8484, -0.5251) (5.8572, -0.53) (5.8659, -0.535) (5.8746, -0.5401) (5.8834, -0.5451) (5.8921, -0.5502) (5.9008, -0.5554) (5.9095, -0.5606) (5.9182, -0.5658) (5.9269, -0.5711) (5.939, -0.5785) (5.9494, -0.585) (5.958, -0.5904) (5.9649, -0.5948) (5.9701, -0.5981) knots 0 0 0 0 0 0 0.014286 0.028571 0.042857 0.057143 0.071429 0.085714 0.1 0.114286 0.128571 0.142857 0.157143 0.171429 0.185714 0.2 0.214286 0.228571 0.242857 0.257143 0.271429 0.285714 0.3 0.314286 0.328571 0.342857 0.357143 0.371429 0.385714 0.4 0.414286 0.428571 0.442857 0.457143 0.471429 0.485714 0.5 0.514286 0.528571 0.542857 0.557143 0.571429 0.585714 0.6 0.614286 0.628571 0.642857 0.657143 0.671429 0.685714 0.7 0.714286 0.728571 0.742857 0.757143 0.771429 0.785714 0.8 0.814286 0.828571 0.842857 0.857143 0.871429 0.885714 0.9 0.914286 0.928571 0.942857 0.957143 1 1 1 1 1 1
  line L43 (5.2789, -0.33) -> (5.3458, -0.3347)
  arc A44 (5.2789, -0.33) -> (5.289, -0.047) centre (0, 0) ccw
  line L44 (5.289, -0.047) -> (5.356, -0.0471)
  spline S44 degree 5 poles (5.356, -0.0471) (5.3579, -0.0471) (5.3616, -0.047) (5.3672, -0.0469) (5.3746, -0.0465) (5.3839, -0.0456) (5.3931, -0.0446) (5.4023, -0.0434) (5.4116, -0.0421) (5.4208, -0.0408) (5.4301, -0.0394) (5.4394, -0.0379) (5.4486, -0.0363) (5.4579, -0.0347) (5.4671, -0.0329) (5.4764, -0.031) (5.4856, -0.029) (5.4949, -0.027) (5.5041, -0.0248) (5.5133, -0.0227) (5.5226, -0.0204) (5.5318, -0.0181) (5.541, -0.0157) (5.5503, -0.0133) (5.5595, -0.0108) (5.5687, -0.0082) (5.5779, -0.0055) (5.5872, -0.0028) (5.5964, -0.0001) (5.6056, 0.0027) (5.6148, 0.0056) (5.624, 0.0085) (5.6332, 0.0115) (5.6424, 0.0146) (5.6516, 0.0177) (5.6608, 0.0208) (5.67, 0.024) (5.6791, 0.0273) (5.6883, 0.0306) (5.6975, 0.034) (5.7067, 0.0374) (5.7158, 0.0409) (5.725, 0.0444) (5.7342, 0.0479) (5.7433, 0.0515) (5.7525, 0.0552) (5.7616, 0.0589) (5.7707, 0.0627) (5.7799, 0.0665) (5.789, 0.0703) (5.7981, 0.0742) (5.8073, 0.0782) (5.8164, 0.0822) (5.8255, 0.0862) (5.8346, 0.0903) (5.8437, 0.0944) (5.8528, 0.0986) (5.8619, 0.1028) (5.871, 0.1071) (5.88, 0.1114) (5.8891, 0.1157) (5.8982, 0.1201) (5.9073, 0.1245) (5.9163, 0.129) (5.9254, 0.1335) (5.9344, 0.1381) (5.9434, 0.1427) (5.9525, 0.1473) (5.9651, 0.1539) (5.9759, 0.1596) (5.985, 0.1644) (5.9922, 0.1683) (5.9976, 0.1712) knots 0 0 0 0 0 0 0.014286 0.028571 0.042857 0.057143 0.071429 0.085714 0.1 0.114286 0.128571 0.142857 0.157143 0.171429 0.185714 0.2 0.214286 0.228571 0.242857 0.257143 0.271429 0.285714 0.3 0.314286 0.328571 0.342857 0.357143 0.371429 0.385714 0.4 0.414286 0.428571 0.442857 0.457143 0.471429 0.485714 0.5 0.514286 0.528571 0.542857 0.557143 0.571429 0.585714 0.6 0.614286 0.628571 0.642857 0.657143 0.671429 0.685714 0.7 0.714286 0.728571 0.742857 0.757143 0.771429 0.785714 0.8 0.814286 0.828571 0.842857 0.857143 0.871429 0.885714 0.9 0.914286 0.928571 0.942857 0.957143 1 1 1 1 1 1
  arc A45 (5.9976, 0.1712) -> (5.9871, 0.3927) centre (0, 0) ccw
  spline S45 degree 5 poles (5.328, 0.5498) (5.3298, 0.5499) (5.3335, 0.5502) (5.3391, 0.5506) (5.3465, 0.5509) (5.3558, 0.5509) (5.3651, 0.5508) (5.3744, 0.5505) (5.3837, 0.5501) (5.3931, 0.5496) (5.4024, 0.5491) (5.4118, 0.5485) (5.4211, 0.5478) (5.4305, 0.547) (5.4399, 0.5461) (5.4493, 0.545) (5.4587, 0.5439) (5.4681, 0.5428) (5.4775, 0.5415) (5.4869, 0.5402) (5.4963, 0.5389) (5.5057, 0.5374) (5.5151, 0.5359) (5.5245, 0.5344) (5.5339, 0.5327) (5.5434, 0.531) (5.5528, 0.5293) (5.5622, 0.5274) (5.5716, 0.5255) (5.5811, 0.5236) (5.5905, 0.5216) (5.5999, 0.5196) (5.6094, 0.5174) (5.6188, 0.5153) (5.6283, 0.5131) (5.6377, 0.5108) (5.6472, 0.5084) (5.6566, 0.5061) (5.6661, 0.5036) (5.6755, 0.5011) (5.685, 0.4986) (5.6944, 0.496) (5.7039, 0.4934) (5.7133, 0.4907) (5.7228, 0.4879) (5.7322, 0.4852) (5.7417, 0.4823) (5.7511, 0.4794) (5.7606, 0.4765) (5.77, 0.4735) (5.7795, 0.4705) (5.7889, 0.4674) (5.7984, 0.4643) (5.8078, 0.4612) (5.8173, 0.458) (5.8267, 0.4547) (5.8362, 0.4514) (5.8456, 0.4481) (5.8551, 0.4447) (5.8645, 0.4412) (5.874, 0.4378) (5.8834, 0.4342) (5.8928, 0.4307) (5.9023, 0.4271) (5.9117, 0.4234) (5.9212, 0.4197) (5.9306, 0.416) (5.94, 0.4122) (5.9532, 0.4069) (5.9645, 0.4022) (5.9739, 0.3983) (5.9815, 0.3951) (5.9871, 0.3927) knots 0 0 0 0 0 0 0.014286 0.028571 0.042857 0.057143 0.071429 0.085714 0.1 0.114286 0.128571 0.142857 0.157143 0.171429 0.185714 0.2 0.214286 0.228571 0.242857 0.257143 0.271429 0.285714 0.3 0.314286 0.328571 0.342857 0.357143 0.371429 0.385714 0.4 0.414286 0.428571 0.442857 0.457143 0.471429 0.485714 0.5 0.514286 0.528571 0.542857 0.557143 0.571429 0.585714 0.6 0.614286 0.628571 0.642857 0.657143 0.671429 0.685714 0.7 0.714286 0.728571 0.742857 0.757143 0.771429 0.785714 0.8 0.814286 0.828571 0.842857 0.857143 0.871429 0.885714 0.9 0.914286 0.928571 0.942857 0.957143 1 1 1 1 1 1
  line L45 (5.2612, 0.5434) -> (5.328, 0.5498)
  arc A46 (5.2612, 0.5434) -> (5.2246, 0.8242) centre (0, 0) ccw
  line L46 (5.2246, 0.8242) -> (5.2907, 0.8352)
  spline S46 degree 5 poles (5.2907, 0.8352) (5.2926, 0.8355) (5.2962, 0.8361) (5.3017, 0.8372) (5.309, 0.8388) (5.3179, 0.8411) (5.3269, 0.8437) (5.3358, 0.8464) (5.3447, 0.8492) (5.3536, 0.852) (5.3625, 0.8549) (5.3714, 0.8579) (5.3803, 0.861) (5.3892, 0.8642) (5.398, 0.8674) (5.4068, 0.8708) (5.4156, 0.8743) (5.4244, 0.8778) (5.4331, 0.8814) (5.4419, 0.8851) (5.4506, 0.8889) (5.4593, 0.8926) (5.4681, 0.8965) (5.4768, 0.9004) (5.4854, 0.9044) (5.4941, 0.9085) (5.5028, 0.9126) (5.5114, 0.9168) (5.5201, 0.9211) (5.5287, 0.9253) (5.5373, 0.9297) (5.5459, 0.9341) (5.5545, 0.9386) (5.563, 0.9431) (5.5716, 0.9477) (5.5801, 0.9523) (5.5887, 0.957) (5.5972, 0.9617) (5.6057, 0.9665) (5.6142, 0.9713) (5.6227, 0.9762) (5.6312, 0.9811) (5.6396, 0.9861) (5.6481, 0.9911) (5.6565, 0.9962) (5.6649, 1.0013) (5.6733, 1.0064) (5.6817, 1.0116) (5.6901, 1.0169) (5.6985, 1.0222) (5.7068, 1.0276) (5.7152, 1.0329) (5.7235, 1.0384) (5.7318, 1.0439) (5.7402, 1.0494) (5.7485, 1.055) (5.7567, 1.0606) (5.765, 1.0662) (5.7733, 1.0719) (5.7815, 1.0777) (5.7898, 1.0834) (5.798, 1.0893) (5.8062, 1.0951) (5.8144, 1.101) (5.8226, 1.107) (5.8307, 1.113) (5.8389, 1.119) (5.847, 1.1251) (5.8584, 1.1336) (5.8682, 1.141) (5.8763, 1.1472) (5.8827, 1.1522) (5.8876, 1.156) knots 0 0 0 0 0 0 0.014286 0.028571 0.042857 0.057143 0.071429 0.085714 0.1 0.114286 0.128571 0.142857 0.157143 0.171429 0.185714 0.2 0.214286 0.228571 0.242857 0.257143 0.271429 0.285714 0.3 0.314286 0.328571 0.342857 0.357143 0.371429 0.385714 0.4 0.414286 0.428571 0.442857 0.457143 0.471429 0.485714 0.5 0.514286 0.528571 0.542857 0.557143 0.571429 0.585714 0.6 0.614286 0.628571 0.642857 0.657143 0.671429 0.685714 0.7 0.714286 0.728571 0.742857 0.757143 0.771429 0.785714 0.8 0.814286 0.828571 0.842857 0.857143 0.871429 0.885714 0.9 0.914286 0.928571 0.942857 0.957143 1 1 1 1 1 1
  arc A47 (5.8876, 1.156) -> (5.8408, 1.3728) centre (0, 0) ccw